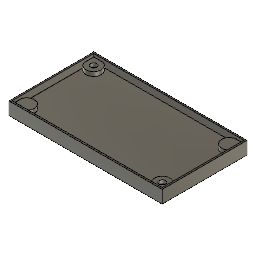
PCB_PDP_TD01_GP08 (Autodesk Fusion 360 archive; units mm, degrees)
design "Socle PlatProt"
Autodesk Fusion 360 part; units mm, degrees
note: some values were not read from the file. Set by a fixed rule: which face or edge a step refers to.
sketch "Sketch1" plane through (0, 0, 0) normal (0, 0, 1) x (1, 0, 0)
  line L0 (20, 63.2) -> (98, 63.2)
  line L1 (98, 63.2) -> (98, 20)
  line L2 (98, 20) -> (20, 20)
  line L3 (20, 20) -> (20, 63.2)
  dimension "d1" = 78
  dimension "d2" = 20
  dimension "d4" = 43.2
  dimension "d5" = 20
  constraint horizontal L0
  constraint vertical L1
  constraint horizontal L2
  constraint vertical L3
  measures "d1" distance of L0.start L0.end
  measures "d2" horizontal distance of origin L2.end
  measures "d4" distance of L0 L2
  measures "d5" vertical distance of origin L2.end
extrude "Extrude4" add sketch "Sketch1" along normal blind 6.6
sketch "Profondeurboite" plane through (0, 0, 6.6) normal (0, 0, 1) x (-1, 0, 0)
  line L0 (-20, -20) -> (-98, -20)
  line L1 (-98, -20) -> (-98, -63.2)
  line L2 (-98, -63.2) -> (-20, -63.2)
  line L3 (-20, -63.2) -> (-20, -20)
  line L4 (-97.2, -20.8) -> (-20.8, -20.8)
  line L5 (-20.8, -20.8) -> (-20.8, -62.4)
  line L6 (-20.8, -62.4) -> (-97.2, -62.4)
  line L7 (-97.2, -62.4) -> (-97.2, -20.8)
  dimension "d20" = 76.4
  dimension "d21" = 41.6
  dimension "d22" = 0.8
  dimension "d23" = 0.8
  constraint horizontal L4
  constraint vertical L5
  constraint horizontal L6
  constraint vertical L7
  measures "d20" distance of L4.start L4.end
  measures "d21" distance of L4 L6
  measures "d22" horizontal distance of L0.end L4.start
  measures "d23" vertical distance of L0.end L4.start
extrude "Extrude6" cut sketch "Profondeurboite" against normal blind 3.6 contours L4 L5 L6 L7
sketch "trous pour ecrous" plane through (0, 0, 0) normal (0, 0, 1) x (1, 0, 0)
  line L0 (20, 20) -> (20, 63.2)
  line L1 (20, 63.2) -> (98, 63.2)
  line L2 (98, 20) -> (20, 20)
  line L3 (98, 63.2) -> (98, 20)
  line L4 (26.0877, 55.85) -> (27.6754, 58.6)
  line L5 (27.6754, 58.6) -> (26.0877, 61.35)
  line L6 (26.0877, 61.35) -> (22.9123, 61.35)
  line L7 (22.9123, 61.35) -> (21.3246, 58.6)
  line L8 (21.3246, 58.6) -> (22.9123, 55.85)
  line L9 (22.9123, 55.85) -> (26.0877, 55.85)
  line L10 (95.0877, 21.85) -> (96.6754, 24.6)
  line L11 (96.6754, 24.6) -> (95.0877, 27.35)
  line L12 (95.0877, 27.35) -> (91.9123, 27.35)
  line L13 (91.9123, 27.35) -> (90.3246, 24.6)
  line L14 (90.3246, 24.6) -> (91.9123, 21.85)
  line L15 (91.9123, 21.85) -> (95.0877, 21.85)
  circle A0 centre (24.5, 58.6) radius 1.6
  circle A1 centre (93.5, 24.6) radius 1.6
  point P0 (24.5, 58.6)
  point P1 (93.5, 24.6)
  dimension "d32" = 2.75
  dimension "d33" = 4.5
  dimension "d34" = 4.6
  dimension "d35" = 2.75
  dimension "d36" = 4.6
  dimension "d37" = 4.5
  dimension "d38" = 3.2
  dimension "d39" = 3.2
  constraint parallel L1 L6
  constraint parallel L2 L15
  constraint coincident P0 A0.centre
  constraint coincident P1 A1.centre
  measures "d32" distance of P0 L9
  measures "d33" distance of L0 P0
  measures "d34" distance of L1 P0
  measures "d35" distance of P1 L15
  measures "d36" distance of L2 P1
  measures "d37" distance of L3 P1
  measures "d38" diameter of A0
  measures "d39" diameter of A1
extrude "Extrude7" cut sketch "trous pour ecrous" along normal blind 3 contours A0 | A1
extrude "Extrude8" cut sketch "trous pour ecrous" along normal blind 2.7 contours L4 L5 L6 L7 L8 L9 | L10 L11 L12 L13 L14 L15
sketch "Extensions decrous" plane through (0, 0, 3) normal (0, 0, 1) x (-1, 0, 0)
  circle A0 centre (-24.5, -58.6) radius 1.6
  circle A1 centre (-93.5, -24.6) radius 1.6
  line L0 (-97.2, -62.4) -> (-20.8, -62.4)
  line L1 (-20.8, -62.4) -> (-20.8, -20.8)
  line L2 (-20.8, -20.8) -> (-97.2, -20.8)
  line L3 (-97.2, -20.8) -> (-97.2, -62.4)
  circle A2 centre (-24.5, -58.6) radius 3.9
  circle A3 centre (-93.5, -24.6) radius 3.9
  circle A4 centre (-93.5, -58.6) radius 3.9
  line L4 (-24.5, -58.6) -> (-97.2, -58.6)
  line L5 (-20, -63.2) -> (-98, -63.2)
  line L6 (-93.5, -24.6) -> (-93.5, -62.4)
  line L7 (-24.5, -58.6) -> (-24.5, -20.8)
  line L8 (-93.5, -24.6) -> (-20.8, -24.6)
  line L9 (-98, -20) -> (-20, -20)
  line L10 (-20, -20) -> (-20, -63.2)
  circle A5 centre (-24.5, -24.6) radius 3.9
  point P0 (-24.5, -58.6)
  point P1 (-93.5, -24.6)
  dimension "d44" = 7.8
  dimension "d45" = 7.8
  dimension "d48" = 7.8
  dimension "d49" = 7.8
  constraint coincident P0 A0.centre
  constraint coincident P1 A1.centre
  constraint coincident L3 L4.end
  constraint parallel L4 L5
  constraint coincident L0 L6.end
  constraint perpendicular L4 L6
  constraint coincident L2 L7.end
  constraint coincident L1 L8.end
  constraint parallel L8 L9
  constraint parallel L7 L10
  constraint coincident A4.centre L6
  constraint coincident A4.centre L4
  constraint coincident L7 A5.centre
  constraint coincident L8 A5.centre
  measures "d44" diameter of A2
  measures "d45" diameter of A3
  measures "d48" diameter of A4
  measures "d49" diameter of A5
extrude "Extrude9" add sketch "Extensions decrous" along normal blind 2 contours A0 L0 L1 A2 L4 L7 | A0 A2 L4 L7 | A1 L2 L3 A3 L6 L8 | A1 A3 L6 L8
extrude "Extrude10" add sketch "Extensions decrous" along normal blind 2 contours L7 L8 A5 | L1 L7 L8 A5 | A4 L4 L6 | L0 A4 L4 L6 | L2 L7 L8 A5 | L1 L2 L7 L8 A5 | L3 A4 L4 L6 | L0 L3 A4 L4 L6
sketch "planDroite" plane through (0, 0, 2.7) normal (0, 0, -1) x (1, 0, 0)
  circle A0 centre (93.5, -24.6) radius 1.6
  line L0 (95.0877, -21.85) -> (91.9123, -21.85)
  line L1 (91.9123, -21.85) -> (90.3246, -24.6)
  line L2 (90.3246, -24.6) -> (91.9123, -27.35)
  line L3 (91.9123, -27.35) -> (95.0877, -27.35)
  line L4 (95.0877, -27.35) -> (96.6754, -24.6)
  line L5 (96.6754, -24.6) -> (95.0877, -21.85)
  line L6 (95.0877, -21.85) -> (95.0877, -27.35)
  line L7 (91.9123, -21.85) -> (91.9123, -27.35)
  line L8 (91.9123, -26.2) -> (95.0877, -26.2)
  line L9 (95.0877, -23) -> (91.9123, -23)
  constraint coincident L0.start L5.end
  constraint coincident L3.end L4.start
  constraint coincident L0.end L1.start
  constraint coincident L2.end L3.start
  constraint coincident L7 L8.start
  constraint coincident L6 L8.end
  constraint perpendicular L6 L8
  constraint coincident L6 L9.start
  constraint coincident L7 L9.end
  constraint tangent A0 L9
  constraint tangent A0 L8
  constraint parallel L8 L9
sketch "PlanGauche" plane through (0, 0, 2.7) normal (0, 0, -1) x (1, 0, 0)
  circle A0 centre (24.5, -58.6) radius 1.6
  line L0 (26.0877, -55.85) -> (22.9123, -55.85)
  line L1 (22.9123, -55.85) -> (21.3246, -58.6)
  line L2 (21.3246, -58.6) -> (22.9123, -61.35)
  line L3 (22.9123, -61.35) -> (26.0877, -61.35)
  line L4 (26.0877, -61.35) -> (27.6754, -58.6)
  line L5 (27.6754, -58.6) -> (26.0877, -55.85)
  line L6 (22.9123, -55.85) -> (22.9123, -61.35)
  line L7 (26.0877, -61.35) -> (26.0877, -55.85)
  line L8 (26.0877, -57) -> (22.9123, -57)
  line L9 (26.0877, -60.2) -> (22.9123, -60.2)
  constraint coincident L0.end L1.start
  constraint coincident L2.end L3.start
  constraint coincident L3.end L4.start
  constraint coincident L0.start L5.end
  constraint coincident L7 L8.start
  constraint coincident L6 L8.end
  constraint perpendicular L6 L8
  constraint coincident L7 L9.start
  constraint coincident L6 L9.end
  constraint perpendicular L6 L9
  constraint tangent A0 L8
  constraint tangent A0 L9
extrude "Extrude11" cut sketch "planDroite" sketch "PlanGauche" against normal blind 0.6 contours A0 L6 L9 | A0 L6 L8 | A0 L7 L9 | A0 L7 L8 of sketch 2 contours A0 L7 L8 | A0 L7 L9 | A0 L6 L8 | A0 L6 L9
extrude "Extrude12" cut sketch "planDroite" sketch "PlanGauche" against normal blind 0.3 contours L0 L6 L7 L9 | L3 L6 L7 L8 of sketch 2 contours L0 L6 L7 L8 | L3 L6 L7 L9
extrude "Extrude13" add 4 faces at (96.4781, 61.785, 3) (96.4781, 21.415, 3) (21.5219, 61.785, 3) (21.5219, 21.415, 3) along direction (0, 0, 1) up to surface end surface through (0, 0, 5) normal (0, 0, 1) offset 0
extrude "Extrude14" add 4 faces at (95.6742, 60.7224, 5) (23.3643, 61.6298, 5) (22.3258, 22.4776, 5) (94.6357, 21.5702, 5) along direction (0, 0, 1) blind 0.1
